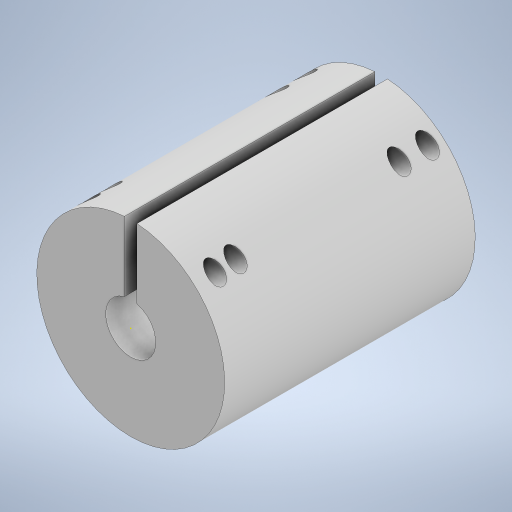
# Autodesk Inventor part: Acoplador de servomotor
Saved by Autodesk Inventor 2024.3 (Build 283343000, 343)
## iProperties
Created: 2025-11-05
Part Number: Acoplador de servomotor
Material: Generic
Document SubType Name: Modeling
Designer: Windows11
Density: 1 g/cm^3
Appearance: Default
Author: Windows11
Autodesk Inventor part; units mm, degrees
ref_plane "YZ Plane" through (0, 0, 0) normal (1, 0, 0) x (0, 1, 0)
ref_plane "XZ Plane" through (0, 0, 0) normal (0, 1, 0) x (-1, 0, 0)
ref_plane "XY Plane" through (0, 0, 0) normal (0, 0, 1) x (1, 0, 0)
sketch "Sketch1" plane through (0, 0, 0) normal (0, 0, 1) x (1, 0, 0)
  circle A0 centre (0, 0) radius 15
  dimension "d0" = 30
  constraints: 1 centre point, 1 coincident
  measures "d0" diameter of A0
extrude "Extrusion1" add sketch "Sketch1" along normal blind 40
sketch "Sketch2" plane through (0, 0, 40) normal (0, 0, 1) x (1, 0, 0)
  circle A0 centre (0, 0) radius 4
  dimension "d3" = 8
  constraints: 1 centre point, 1 coincident
  measures "d3" diameter of A0
extrude "Extrusion2" cut sketch "Sketch2" against normal blind 40
sketch "Sketch3" plane through (0, 0, 40) normal (0, 0, 1) x (1, 0, 0)
  circle A0 centre (0, 0) radius 4 projected
  circle A1 centre (0, 0) radius 15 projected
  line L0 (0, 15) -> (1, 15)
  line L1 (0, 15) -> (-1, 15)
  line L2 (-0.0081, 4) -> (0.9843, 3.877)
  line L3 (-0.0081, 4) -> (-1, 3.873)
  line L4 (-1, 3.873) -> (-1, 15)
  line L5 (0.9843, 3.877) -> (1, 15)
  dimension "d8" = 1
  dimension "d9" = 1
  dimension "d10" = 1
  dimension "d11" = 1
  constraints: 12 end point, 3 horizontal, 3 point on circle, 1 vertical, 1 vertical alignment, 1 other
  measures "d8" distance of L0.start L0.end
  measures "d9" distance of L0.start L1.end
  measures "d10" distance of L2.start L2.end
  measures "d11" distance of L2.start L3.end
extrude "Extrusion3" cut sketch "Sketch3" against normal blind 40 contours L2 A0 | A0 L4 A1 L5 | A0 L3 | A1 L0 L5 | L4 L1 A1 picked at (-0.339, 7.6568)
sketch "Sketch4" plane through (0, 0, 40) normal (0, 0, 1) x (1, 0, 0)
  point P0 (0, 0)
sketch "Sketch5" plane through (1, 14.9666, 0) normal (-1, 0.0014, 0) x (0, 0, 1)
  point P0 (0, -14.968)
sketch "Sketch6" plane through (1, 14.9666, 0) normal (-1, 0.0014, 0) x (0, 0, 1)
  circle A0 centre (36.6199, -3.9195) radius 1.25
  point P0 (0, -14.968)
  dimension "d14" = 2.5
  constraints: 1 centre point
  measures "d14" diameter of A0
extrude "Extrusion4" cut sketch "Sketch6" against normal blind 15
sketch "Sketch7" plane through (1, 14.9666, 0) normal (-1, 0.0014, 0) x (0, 0, 1)
  circle A0 centre (33.2561, -3.8302) radius 1.25
  point P0 (0, -14.968)
  dimension "d17" = 2.5
  constraints: 1 centre point
  measures "d17" diameter of A0
extrude "Extrusion5" cut sketch "Sketch7" against normal blind 15
sketch "Sketch8" plane through (1, 14.9666, 0) normal (-1, 0.0014, 0) x (0, 0, 1)
  circle A0 centre (6.8967, -3.6366) radius 1.25
  circle A1 centre (2.3686, -3.6366) radius 1.25
  point P0 (0, -14.968)
  dimension "d20" = 2.5
  dimension "d21" = 2.5
  constraints: 2 centre point
  measures "d20" diameter of A0
  measures "d21" diameter of A1
extrude "Extrusion6" cut sketch "Sketch8" against normal blind 30
sketch "Sketch9" plane through (-1, 3.873, 40) normal (1, 0, 0) x (0, 0, -1)
  point P0 (40, -3.873)
sketch "Sketch10" plane through (-1, 3.873, 40) normal (1, 0, 0) x (0, 0, -1)
  ellipse E0 centre (33.1033, 7.4571) end of major axis (31.8533, 7.4571) minor radius 1.25 projected
  circle A0 centre (33.1033, 7.4571) radius 1.25
  ellipse E1 centre (37.6314, 7.4571) end of major axis (36.3814, 7.4571) minor radius 1.25 projected
  circle A1 centre (37.6314, 7.4571) radius 1.25
  ellipse E2 centre (6.7439, 7.2634) end of major axis (5.4939, 7.2634) minor radius 1.25 projected
  circle A2 centre (6.7439, 7.2634) radius 1.25
  ellipse E3 centre (3.3801, 7.1742) end of major axis (2.1301, 7.1742) minor radius 1.25 projected
  circle A3 centre (3.3801, 7.1742) radius 1.25
  point P0 (40, -3.873)
  dimension "d24" = 2.5
  dimension "d25" = 2.5
  dimension "d26" = 2.5
  dimension "d27" = 2.5
  constraints: 4 centre point, 4 coincident, 4 other
  measures "d24" diameter of A0
  measures "d25" diameter of A1
  measures "d26" diameter of A2
  measures "d27" diameter of A3
extrude "Extrusion7" cut sketch "Sketch10" against normal blind 30
body "Solid1"
